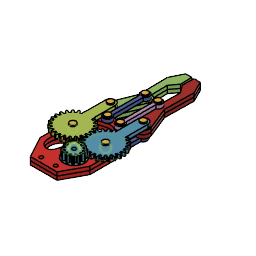
ARC Robotic-Gripper (Autodesk Fusion 360 design; units mm, degrees)
part number: 2026-08-30-15-38-19-867
part number: 2026-08-30-16-06-25-196
part number: 2026-08-30-16-15-02-917
part number: 2026-08-30-20-55-51-300
description: Spur Gear; Module: 1.125; Num Teeth: 24; Pressure Angle: 20.0; Backlash: 0.00 mm
part number: 2026-08-30-21-05-14-429
part number: 2026-08-30-21-11-26-364
part number: 2026-08-30-22-11-41-615
description: Spur Gear; Module: 1.1; Num Teeth: 12; Pressure Angle: 20.0; Backlash: 0.00 mm
part number: 2026-08-30-22-17-12-966
Autodesk Fusion 360 part; units mm, degrees
note: some values were not read from the file. Chosen so that the rebuilt part matches the saved one: a direction. Set by a fixed rule: which sketch regions a step uses.
(part 1 of 8)
sketch "Sketch1" plane through (0, 0, 0) normal (0, 1, 0) x (1, 0, 0)
  line L0 (0, -5) -> (22, -5)
  arc A0 (22, -5) -> (22, 5) centre (22, 0) ccw
  line L1 (22, 5) -> (0, 5)
  arc A1 (0, 5) -> (0, -5) centre (0, 0) ccw
  line L2 (0, 0) -> (22, 0) construction
  circle A2 centre (0, 0) radius 1.5
  line L3 (20.05, 5) -> (51.3472, 18.2849)
  line L4 (51.3472, 18.2849) -> (55.3871, 8.7674)
  line L5 (55.3871, 8.7674) -> (24.4042, -4.384)
  line L6 (42.1568, 14.3838) -> (53.3671, 13.5261)
  line L7 (26.6766, 1.769) -> (39, 7)
  line L8 (39, 7) -> (46.5562, 5.0189)
  circle A3 centre (22, 0) radius 1.5
  dimension "d1" = 22
  dimension "d2" = 5
  dimension "d3" = 3
  dimension "d4" = 157
  dimension "d5" = 34
  dimension "d6" = 1.95
  dimension "d7" = 3
  constraint tangent L0 A0
  constraint tangent A0 L1
  constraint parallel L0 L1
  constraint tangent L1 A1
  constraint tangent L0 A1
  constraint horizontal L2
  constraint coincident A1.centre L2.start
  constraint coincident L1 L3.start
  constraint perpendicular L3 L4
  constraint coincident A0 L5.end
  constraint perpendicular L4 L5
  constraint coincident L3 L6.start
  constraint midpoint L4 L6.end
  constraint coincident A0 L7.start
  constraint perpendicular L4 L7
  constraint coincident L5 L8.end
  constraint concentric A0 A3
  measures "d1" distance of A1.centre A0.centre
  measures "d2" radius of A1
  measures "d3" diameter of A2
  measures "d4" angle of L1 L3
  measures "d5" distance of L3.start L3.end
  measures "d6" horizontal distance of A0.centre L3.start
  measures "d7" diameter of A3
extrude "Extrude1" add sketch "Sketch1" along normal blind 3 contours L0 A0 L1 A1 | A0 L1 L3 L4 L5 L6 L7 L8 makes body 1
copy_body "Body->Comp1" bodies 1 removing the originals makes body 2 in component "Component"
sketch "Sketch2" plane through (0, 0, 0) normal (0, 1, 0) x (1, 0, 0)
  circle A0 centre (2, 10) radius 1.5
  circle A1 centre (2, 10) radius 3.5
  circle A2 centre (33, 10) radius 3.5
  circle A3 centre (33, 10) radius 1.5
  line L0 (2, 10) -> (33, 10)
  line L1 (5.1623, 11.5) -> (29.8377, 11.5)
  line L2 (5.1623, 8.5) -> (29.8377, 8.5)
  dimension "d11" = 7
  dimension "d12" = 3
  dimension "d14" = 7
  dimension "d15" = 3
  dimension "d16" = 31
  dimension "d17" = 1.5
  constraint concentric A0 A1
  constraint concentric A2 A3
  constraint coincident A0.centre A1.centre
  constraint coincident A2.centre A3.centre
  constraint horizontal L0
  constraint coincident A1 L1.start
  constraint coincident A2 L1.end
  constraint parallel L0 L1
  constraint symmetric L0 L1.start L2.start
  constraint symmetric L0 L1.end L2.end
  measures "d11" diameter of A1
  measures "d12" diameter of A0
  measures "d14" diameter of A2
  measures "d15" diameter of A3
  measures "d16" distance of A0.centre A2.centre
  measures "d17" distance of L0 L1
extrude "Extrude1'" add sketch "Sketch2" along normal blind 3 separate body makes body 3 in component "Component'"
sketch "Sketch3" plane through (0, 0, 0) normal (0, 1, 0) x (1, 0, 0)
  line L0 (0, 0) -> (0, 62) construction
  line L1 (0, 62) -> (-7.9898, 62)
  line L2 (-7.9898, 62) -> (-20.5, 47.8997)
  line L3 (-20.5, 47.8997) -> (-20.5, 17.5997)
  line L4 (-20.5, 17.5997) -> (-11, 0)
  line L5 (-11, 0) -> (0, 0)
  circle A0 centre (-6, 4) radius 1.5
  circle A1 centre (-13.5, 37.5997) radius 1.5
  circle A2 centre (-5.2398, 58) radius 1.5
  circle A3 centre (6, 4) radius 1.5
  line L6 (20.5, 47.8997) -> (20.5, 17.5997)
  circle A4 centre (5.2398, 58) radius 1.5
  circle A5 centre (13.5, 37.5997) radius 1.5
  line L7 (20.5, 17.5997) -> (11, 0)
  line L8 (11, 0) -> (0, 0)
  line L9 (0, 62) -> (7.9898, 62)
  line L10 (7.9898, 62) -> (20.5, 47.8997)
  circle A6 centre (7.5, 17.5997) radius 8.5
  line L11 (20.5, 17.5997) -> (2, 17.5997) construction
  dimension "d20" = 62
  dimension "d21" = 11
  dimension "d22" = 20
  dimension "d23" = 20.5
  dimension "d24" = 30.3
  dimension "d25" = 18.85
  dimension "d26" = 3
  dimension "d27" = 3
  dimension "d28" = 3
  dimension "d29" = 4
  dimension "d30" = 2.75
  dimension "d31" = 10.3
  dimension "d32" = 7
  dimension "d33" = 6
  dimension "d34" = 4
  dimension "d35" = 17
  dimension "d36" = 13
  constraint coincident L0.start L5.end
  constraint vertical L0
  constraint perpendicular L0 L1
  constraint perpendicular L1 L3
  constraint perpendicular L0 L5
  constraint symmetric L5.end L0 L8.end
  constraint symmetric L1.start L0 L9.start
  constraint symmetric L0 L1.end L9.end
  constraint symmetric L0 L2.end L6.start
  constraint symmetric L0 L3.end L6.end
  constraint symmetric L0 L4.end L7.end
  constraint symmetric L0 A0 A3
  constraint symmetric L0 A1 A5
  constraint symmetric L0 A2 A4
  constraint perpendicular L6 L11
  measures "d20" distance of L0.start L0.end
  measures "d21" distance of L0.start L4.end
  measures "d22" distance of L3.end L4.end
  measures "d23" distance of L0 L3
  measures "d24" distance of L2.end L3.end
  measures "d25" distance of L1.end L2.end
  measures "d26" diameter of A0
  measures "d27" diameter of A1
  measures "d28" diameter of A2
  measures "d29" distance of L1 A2.centre
  measures "d30" horizontal distance of L1.end A2.centre
  measures "d31" vertical distance of L2.end A1.centre
  measures "d32" distance of L3 A1.centre
  measures "d33" distance of L0 A0.centre
  measures "d34" distance of L5 A0.centre
  measures "d35" diameter of A6
  measures "d36" distance of L6.end A6.centre
extrude "Extrude1''" add sketch "Sketch3" along normal blind 3 separate body makes body 4 in component "Component''"
sketch "Sketch4" plane through (0, 3, 0) normal (0, 1, 0) x (-1, 0, 0)
  circle A0 centre (13.5, -37.5997) radius 1.5
  circle A1 centre (-13.5, -37.5997) radius 1.5
  circle A2 centre (5.2398, -58) radius 1.5
  circle A3 centre (-5.2398, -58) radius 1.5
  circle A4 centre (-7.5, -17.5997) radius 8.5
  circle A5 centre (-6, -4) radius 1.5
  circle A6 centre (6, -4) radius 1.5
  line L0 (-7.9898, -62) -> (7.9898, -62)
  line L1 (7.9898, -62) -> (20.5, -47.8997)
  line L2 (20.5, -47.8997) -> (20.5, -17.5997)
  line L3 (20.5, -17.5997) -> (11, 0)
  line L4 (11, 0) -> (-11, 0)
  line L5 (-11, 0) -> (-20.5, -17.5997)
  line L6 (-20.5, -17.5997) -> (-20.5, -47.8997)
  line L7 (-20.5, -47.8997) -> (-7.9898, -62)
  spline S0 degree 5 poles (-5.4336, -53.3907) (-5.0466, -53.6541) (-4.2829, -54.1428) (-3.1766, -54.7552) (-1.7949, -55.3213) (-0.1877, -55.6395) (1.3743, -55.6316) (2.9743, -55.3768) (4.672, -54.9534) (6.4712, -54.4196) (8.2906, -53.797) (9.9982, -53.0839) (11.4425, -52.2666) (12.4861, -51.3325) (13.0351, -50.2808) (13.0781, -49.1379) (12.6944, -47.958) (12.0103, -46.799) (11.1693, -45.705) (10.2934, -44.6837) (9.4576, -43.6945) (8.7075, -42.6752) (8.0713, -41.564) (7.5718, -40.321) (7.2426, -38.9561) (7.1252, -37.5229) (7.2563, -36.0942) (7.6582, -34.7424) (8.3281, -33.5194) (9.2262, -32.434) (10.2859, -31.4594) (11.4259, -30.5457) (12.5628, -29.6303) (13.6225, -28.649) (14.5534, -27.5475) (15.3216, -26.2861) (15.9046, -24.8443) (16.2852, -23.226) (16.4461, -21.4627) (16.3624, -19.621) (16.0068, -17.7946) (15.3609, -16.0912) (14.4242, -14.6215) (13.2244, -13.4867) (11.8261, -12.7674) (10.3439, -12.5104) (8.9154, -12.7294) (7.6684, -13.407) (6.6915, -14.497) (5.9989, -15.9255) (5.5123, -17.5946) (5.1029, -19.3938) (4.6229, -21.2096) (3.9421, -22.9364) (2.9802, -24.4864) (1.7452, -25.8008) (0.3576, -26.858) (-1.0142, -27.6679) (-2.2075, -28.2677) (-3.1243, -28.7169) (-3.7864, -29.0927) (-4.3954, -29.4854) (-5.191, -29.9812) (-6.3187, -30.6456) (-7.6675, -31.5043) (-8.9566, -32.5465) (-9.8678, -33.7315) (-10.1614, -34.9951) (-9.7992, -36.2553) (-9.0659, -37.4185) (-8.3987, -38.4052) (-8.218, -39.1757) (-8.7535, -39.7561) (-9.8832, -40.2621) (-11.2724, -40.8519) (-12.505, -41.6801) (-13.2098, -42.8549) (-13.2068, -44.3863) (-12.4853, -46.202) (-11.1517, -48.176) (-9.3881, -50.1522) (-7.8027, -51.6062) (-6.6047, -52.5623) (-5.8205, -53.1273) (-5.4336, -53.3907) knots 0 0 0 0 0 0 0.0125 0.025 0.0375 0.05 0.0625 0.075 0.0875 0.1 0.1125 0.125 0.1375 0.15 0.1625 0.175 0.1875 0.2 0.2125 0.225 0.2375 0.25 0.2625 0.275 0.2875 0.3 0.3125 0.325 0.3375 0.35 0.3625 0.375 0.3875 0.4 0.4125 0.425 0.4375 0.45 0.4625 0.475 0.4875 0.5 0.5125 0.525 0.5375 0.55 0.5625 0.575 0.5875 0.6 0.6125 0.625 0.6375 0.65 0.6625 0.675 0.6875 0.7 0.7125 0.725 0.7375 0.75 0.7625 0.775 0.7875 0.8 0.8125 0.825 0.8375 0.85 0.8625 0.875 0.8875 0.9 0.9125 0.925 0.9375 0.95 0.9625 0.975 0.9875 1 1 1 1 1 1
  point P0 (4.6067, -54.9499)
  point P1 (12.7571, -50.674)
  point P2 (11.3396, -45.9491)
  point P3 (7.9141, -41.1061)
  point P4 (7.796, -34.6095)
  point P5 (12.639, -29.5303)
  point P6 (16.3007, -22.6793)
  point P7 (12.9933, -13.4658)
  point P8 (6.9691, -14.2927)
  point P9 (3.0711, -24.2148)
  point P10 (-3.0711, -28.7034)
  point P11 (-5.4336, -30.1209)
  point P12 (-10, -35)
  point P13 (-8.3866, -39.0981)
  point P14 (-12.5208, -41.933)
extrude "Extrude2" cut sketch "Sketch4" against normal blind 5 contours S0 bodies 4 in component "Component''"
sketch "Base Circle" plane through (0, 0, 0) normal (0, 0, 1) x (1, 0, 0) in component "Spur Gear 24 teeth"
  circle A0 centre (0, 0) radius 12.1984
  circle A1 centre (0, 0) radius 1.5
extrude "Extrude1'''" add sketch "Base Circle" along normal blind 3 separate body makes body 5 in component "Spur Gear 24 teeth"
sketch "Gear Tooth" plane through (0, 0, 0) normal (0, 0, 1) x (1, 0, 0) in component "Spur Gear 24 teeth"
  spline S0 degree 5 poles (12.6449, -1.0183) (12.6506, -1.0187) (12.6618, -1.0195) (12.6788, -1.0202) (12.7014, -1.0204) (12.7297, -1.0195) (12.758, -1.0178) (12.7864, -1.0156) (12.8147, -1.0131) (12.8431, -1.0105) (12.8715, -1.0076) (12.8999, -1.0045) (12.9284, -1.0011) (12.9568, -0.9973) (12.9852, -0.9932) (13.0137, -0.9886) (13.0421, -0.9838) (13.0705, -0.9787) (13.099, -0.9733) (13.1274, -0.9678) (13.1559, -0.962) (13.1843, -0.956) (13.2127, -0.9498) (13.2412, -0.9433) (13.2696, -0.9366) (13.298, -0.9297) (13.3264, -0.9226) (13.3549, -0.9152) (13.3833, -0.9076) (13.4117, -0.8999) (13.4401, -0.8919) (13.4684, -0.8838) (13.4968, -0.8754) (13.5252, -0.8669) (13.5535, -0.8581) (13.5819, -0.8492) (13.6102, -0.8401) (13.6385, -0.8308) (13.6669, -0.8214) (13.6952, -0.8117) (13.7234, -0.8019) (13.7517, -0.7919) (13.78, -0.7817) (13.8082, -0.7714) (13.8365, -0.7609) (13.8647, -0.7502) (13.8929, -0.7393) (13.9211, -0.7283) (13.9492, -0.7171) (13.9774, -0.7058) (14.0055, -0.6943) (14.0337, -0.6826) (14.0618, -0.6708) (14.0898, -0.6588) (14.1179, -0.6467) (14.146, -0.6344) (14.174, -0.6219) (14.202, -0.6093) (14.23, -0.5966) (14.2579, -0.5837) (14.2859, -0.5706) (14.3138, -0.5574) (14.3417, -0.544) (14.3696, -0.5305) (14.3975, -0.5169) (14.4253, -0.5031) (14.4531, -0.4891) (14.4809, -0.4751) (14.5087, -0.4608) (14.5364, -0.4465) (14.5641, -0.4319) (14.5863, -0.4202) (14.6029, -0.4114) (14.6139, -0.4054) (14.6195, -0.4024) knots 0 0 0 0 0 0 0.01428571 0.02857143 0.04285714 0.05714286 0.07142857 0.08571429 0.1 0.11428571 0.12857143 0.14285714 0.15714286 0.17142857 0.18571429 0.2 0.21428571 0.22857143 0.24285714 0.25714286 0.27142857 0.28571429 0.3 0.31428571 0.32857143 0.34285714 0.35714286 0.37142857 0.38571429 0.4 0.41428571 0.42857143 0.44285714 0.45714286 0.47142857 0.48571429 0.5 0.51428571 0.52857143 0.54285714 0.55714286 0.57142857 0.58571429 0.6 0.61428571 0.62857143 0.64285714 0.65714286 0.67142857 0.68571429 0.7 0.71428571 0.72857143 0.74285714 0.75714286 0.77142857 0.78571429 0.8 0.81428571 0.82857143 0.84285714 0.85714286 0.87142857 0.88571429 0.9 0.91428571 0.92857143 0.94285714 0.95714286 0.97142857 0.98571429 1 1 1 1 1 1
  spline S1 degree 5 poles (12.6449, 1.0183) (12.6506, 1.0187) (12.6618, 1.0195) (12.6788, 1.0202) (12.7014, 1.0204) (12.7297, 1.0195) (12.758, 1.0178) (12.7864, 1.0156) (12.8147, 1.0131) (12.8431, 1.0105) (12.8715, 1.0076) (12.8999, 1.0045) (12.9284, 1.0011) (12.9568, 0.9973) (12.9852, 0.9932) (13.0137, 0.9886) (13.0421, 0.9838) (13.0705, 0.9787) (13.099, 0.9733) (13.1274, 0.9678) (13.1559, 0.962) (13.1843, 0.956) (13.2127, 0.9498) (13.2412, 0.9433) (13.2696, 0.9366) (13.298, 0.9297) (13.3264, 0.9226) (13.3549, 0.9152) (13.3833, 0.9076) (13.4117, 0.8999) (13.4401, 0.8919) (13.4684, 0.8838) (13.4968, 0.8754) (13.5252, 0.8669) (13.5535, 0.8581) (13.5819, 0.8492) (13.6102, 0.8401) (13.6385, 0.8308) (13.6669, 0.8214) (13.6952, 0.8117) (13.7234, 0.8019) (13.7517, 0.7919) (13.78, 0.7817) (13.8082, 0.7714) (13.8365, 0.7609) (13.8647, 0.7502) (13.8929, 0.7393) (13.9211, 0.7283) (13.9492, 0.7171) (13.9774, 0.7058) (14.0055, 0.6943) (14.0337, 0.6826) (14.0618, 0.6708) (14.0898, 0.6588) (14.1179, 0.6467) (14.146, 0.6344) (14.174, 0.6219) (14.202, 0.6093) (14.23, 0.5966) (14.2579, 0.5837) (14.2859, 0.5706) (14.3138, 0.5574) (14.3417, 0.544) (14.3696, 0.5305) (14.3975, 0.5169) (14.4253, 0.5031) (14.4531, 0.4891) (14.4809, 0.4751) (14.5087, 0.4608) (14.5364, 0.4465) (14.5641, 0.4319) (14.5863, 0.4202) (14.6029, 0.4114) (14.6139, 0.4054) (14.6195, 0.4024) knots 0 0 0 0 0 0 0.01428571 0.02857143 0.04285714 0.05714286 0.07142857 0.08571429 0.1 0.11428571 0.12857143 0.14285714 0.15714286 0.17142857 0.18571429 0.2 0.21428571 0.22857143 0.24285714 0.25714286 0.27142857 0.28571429 0.3 0.31428571 0.32857143 0.34285714 0.35714286 0.37142857 0.38571429 0.4 0.41428571 0.42857143 0.44285714 0.45714286 0.47142857 0.48571429 0.5 0.51428571 0.52857143 0.54285714 0.55714286 0.57142857 0.58571429 0.6 0.61428571 0.62857143 0.64285714 0.65714286 0.67142857 0.68571429 0.7 0.71428571 0.72857143 0.74285714 0.75714286 0.77142857 0.78571429 0.8 0.81428571 0.82857143 0.84285714 0.85714286 0.87142857 0.88571429 0.9 0.91428571 0.92857143 0.94285714 0.95714286 0.97142857 0.98571429 1 1 1 1 1 1
  arc A0 (14.6195, -0.4024) -> (14.6195, 0.4024) centre (0, 0) ccw
  line L0 (12.149, -0.9783) -> (12.6449, -1.0183)
  line L1 (12.149, 0.9783) -> (12.6449, 1.0183)
  line L2 (12.149, -0.9783) -> (12.149, 0.9783)
  point P0 (12.7841, -1.0157)
  point P1 (12.9241, -1.0016)
  point P2 (13.0647, -0.9797)
  point P3 (13.2057, -0.9513)
  point P4 (13.3469, -0.9172)
  point P5 (13.4884, -0.8779)
  point P6 (13.63, -0.8336)
  point P7 (13.7716, -0.7847)
  point P8 (13.9132, -0.7313)
  point P9 (14.0548, -0.6737)
  point P10 (14.1963, -0.6119)
  point P11 (14.3376, -0.546)
  point P12 (14.4787, -0.4761)
  point P13 (12.7841, 1.0157)
  point P14 (12.9241, 1.0016)
  point P15 (13.0647, 0.9797)
  point P16 (13.2057, 0.9513)
  point P17 (13.3469, 0.9172)
  point P18 (13.4884, 0.8779)
  point P19 (13.63, 0.8336)
  point P20 (13.7716, 0.7847)
  point P21 (13.9132, 0.7313)
  point P22 (14.0548, 0.6737)
  point P23 (14.1963, 0.6119)
  point P24 (14.3376, 0.546)
  point P25 (14.4787, 0.4761)
extrude "Extrude2'" add sketch "Gear Tooth" along normal blind 3 bodies 5 in component "Spur Gear 24 teeth"
fillet "Fillet1" radius 0.1 2 edges at (12.159, -0.9791, 1.5) (12.159, 0.9791, 1.5) on bodies 5 in component "Spur Gear 24 teeth"
pattern_circular "C-Pattern1" count 24 over 360 about axis through (0, 0, 0) along (0, 0, 1) of "Extrude2'", "Fillet1" in component "Spur Gear 24 teeth"
sketch "Diametrial Pitch Circle" plane through (0, 0, 0) normal (0, 0, 1) x (1, 0, 0) in component "Spur Gear 24 teeth"
  circle A0 centre (0, 0) radius 13.5 construction
sketch "Base Circle (2)" plane through (0, 0, 0) normal (0, 0, 1) x (1, 0, 0) in component "Spur Gear 24 teeth (1)"
  circle A0 centre (0, 0) radius 12.1984
  circle A1 centre (0, 0) radius 1.5
extrude "Extrude1''''" add sketch "Base Circle (2)" along normal blind 3 separate body makes body 6 in component "Spur Gear 24 teeth (1)"
sketch "Gear Tooth (2)" plane through (0, 0, 0) normal (0, 0, 1) x (1, 0, 0) in component "Spur Gear 24 teeth (1)"
  spline S0 degree 5 poles (12.6449, -1.0183) (12.6506, -1.0187) (12.6618, -1.0195) (12.6788, -1.0202) (12.7014, -1.0204) (12.7297, -1.0195) (12.758, -1.0178) (12.7864, -1.0156) (12.8147, -1.0131) (12.8431, -1.0105) (12.8715, -1.0076) (12.8999, -1.0045) (12.9284, -1.0011) (12.9568, -0.9973) (12.9852, -0.9932) (13.0137, -0.9886) (13.0421, -0.9838) (13.0705, -0.9787) (13.099, -0.9733) (13.1274, -0.9678) (13.1559, -0.962) (13.1843, -0.956) (13.2127, -0.9498) (13.2412, -0.9433) (13.2696, -0.9366) (13.298, -0.9297) (13.3264, -0.9226) (13.3549, -0.9152) (13.3833, -0.9076) (13.4117, -0.8999) (13.4401, -0.8919) (13.4684, -0.8838) (13.4968, -0.8754) (13.5252, -0.8669) (13.5535, -0.8581) (13.5819, -0.8492) (13.6102, -0.8401) (13.6385, -0.8308) (13.6669, -0.8214) (13.6952, -0.8117) (13.7234, -0.8019) (13.7517, -0.7919) (13.78, -0.7817) (13.8082, -0.7714) (13.8365, -0.7609) (13.8647, -0.7502) (13.8929, -0.7393) (13.9211, -0.7283) (13.9492, -0.7171) (13.9774, -0.7058) (14.0055, -0.6943) (14.0337, -0.6826) (14.0618, -0.6708) (14.0898, -0.6588) (14.1179, -0.6467) (14.146, -0.6344) (14.174, -0.6219) (14.202, -0.6093) (14.23, -0.5966) (14.2579, -0.5837) (14.2859, -0.5706) (14.3138, -0.5574) (14.3417, -0.544) (14.3696, -0.5305) (14.3975, -0.5169) (14.4253, -0.5031) (14.4531, -0.4891) (14.4809, -0.4751) (14.5087, -0.4608) (14.5364, -0.4465) (14.5641, -0.4319) (14.5863, -0.4202) (14.6029, -0.4114) (14.6139, -0.4054) (14.6195, -0.4024) knots 0 0 0 0 0 0 0.01428571 0.02857143 0.04285714 0.05714286 0.07142857 0.08571429 0.1 0.11428571 0.12857143 0.14285714 0.15714286 0.17142857 0.18571429 0.2 0.21428571 0.22857143 0.24285714 0.25714286 0.27142857 0.28571429 0.3 0.31428571 0.32857143 0.34285714 0.35714286 0.37142857 0.38571429 0.4 0.41428571 0.42857143 0.44285714 0.45714286 0.47142857 0.48571429 0.5 0.51428571 0.52857143 0.54285714 0.55714286 0.57142857 0.58571429 0.6 0.61428571 0.62857143 0.64285714 0.65714286 0.67142857 0.68571429 0.7 0.71428571 0.72857143 0.74285714 0.75714286 0.77142857 0.78571429 0.8 0.81428571 0.82857143 0.84285714 0.85714286 0.87142857 0.88571429 0.9 0.91428571 0.92857143 0.94285714 0.95714286 0.97142857 0.98571429 1 1 1 1 1 1
  spline S1 degree 5 poles (12.6449, 1.0183) (12.6506, 1.0187) (12.6618, 1.0195) (12.6788, 1.0202) (12.7014, 1.0204) (12.7297, 1.0195) (12.758, 1.0178) (12.7864, 1.0156) (12.8147, 1.0131) (12.8431, 1.0105) (12.8715, 1.0076) (12.8999, 1.0045) (12.9284, 1.0011) (12.9568, 0.9973) (12.9852, 0.9932) (13.0137, 0.9886) (13.0421, 0.9838) (13.0705, 0.9787) (13.099, 0.9733) (13.1274, 0.9678) (13.1559, 0.962) (13.1843, 0.956) (13.2127, 0.9498) (13.2412, 0.9433) (13.2696, 0.9366) (13.298, 0.9297) (13.3264, 0.9226) (13.3549, 0.9152) (13.3833, 0.9076) (13.4117, 0.8999) (13.4401, 0.8919) (13.4684, 0.8838) (13.4968, 0.8754) (13.5252, 0.8669) (13.5535, 0.8581) (13.5819, 0.8492) (13.6102, 0.8401) (13.6385, 0.8308) (13.6669, 0.8214) (13.6952, 0.8117) (13.7234, 0.8019) (13.7517, 0.7919) (13.78, 0.7817) (13.8082, 0.7714) (13.8365, 0.7609) (13.8647, 0.7502) (13.8929, 0.7393) (13.9211, 0.7283) (13.9492, 0.7171) (13.9774, 0.7058) (14.0055, 0.6943) (14.0337, 0.6826) (14.0618, 0.6708) (14.0898, 0.6588) (14.1179, 0.6467) (14.146, 0.6344) (14.174, 0.6219) (14.202, 0.6093) (14.23, 0.5966) (14.2579, 0.5837) (14.2859, 0.5706) (14.3138, 0.5574) (14.3417, 0.544) (14.3696, 0.5305) (14.3975, 0.5169) (14.4253, 0.5031) (14.4531, 0.4891) (14.4809, 0.4751) (14.5087, 0.4608) (14.5364, 0.4465) (14.5641, 0.4319) (14.5863, 0.4202) (14.6029, 0.4114) (14.6139, 0.4054) (14.6195, 0.4024) knots 0 0 0 0 0 0 0.01428571 0.02857143 0.04285714 0.05714286 0.07142857 0.08571429 0.1 0.11428571 0.12857143 0.14285714 0.15714286 0.17142857 0.18571429 0.2 0.21428571 0.22857143 0.24285714 0.25714286 0.27142857 0.28571429 0.3 0.31428571 0.32857143 0.34285714 0.35714286 0.37142857 0.38571429 0.4 0.41428571 0.42857143 0.44285714 0.45714286 0.47142857 0.48571429 0.5 0.51428571 0.52857143 0.54285714 0.55714286 0.57142857 0.58571429 0.6 0.61428571 0.62857143 0.64285714 0.65714286 0.67142857 0.68571429 0.7 0.71428571 0.72857143 0.74285714 0.75714286 0.77142857 0.78571429 0.8 0.81428571 0.82857143 0.84285714 0.85714286 0.87142857 0.88571429 0.9 0.91428571 0.92857143 0.94285714 0.95714286 0.97142857 0.98571429 1 1 1 1 1 1
  arc A0 (14.6195, -0.4024) -> (14.6195, 0.4024) centre (0, 0) ccw
  line L0 (12.149, -0.9783) -> (12.6449, -1.0183)
  line L1 (12.149, 0.9783) -> (12.6449, 1.0183)
  line L2 (12.149, -0.9783) -> (12.149, 0.9783)
  point P0 (12.7841, -1.0157)
  point P1 (12.9241, -1.0016)
  point P2 (13.0647, -0.9797)
  point P3 (13.2057, -0.9513)
  point P4 (13.3469, -0.9172)
  point P5 (13.4884, -0.8779)
  point P6 (13.63, -0.8336)
  point P7 (13.7716, -0.7847)
  point P8 (13.9132, -0.7313)
  point P9 (14.0548, -0.6737)
  point P10 (14.1963, -0.6119)
  point P11 (14.3376, -0.546)
  point P12 (14.4787, -0.4761)
  point P13 (12.7841, 1.0157)
  point P14 (12.9241, 1.0016)
  point P15 (13.0647, 0.9797)
  point P16 (13.2057, 0.9513)
  point P17 (13.3469, 0.9172)
  point P18 (13.4884, 0.8779)
  point P19 (13.63, 0.8336)
  point P20 (13.7716, 0.7847)
  point P21 (13.9132, 0.7313)
  point P22 (14.0548, 0.6737)
  point P23 (14.1963, 0.6119)
  point P24 (14.3376, 0.546)
  point P25 (14.4787, 0.4761)
extrude "Extrude2''" add sketch "Gear Tooth (2)" along normal blind 3 bodies 6 in component "Spur Gear 24 teeth (1)"
fillet "Fillet1'" radius 0.1 2 edges at (12.159, -0.9791, 1.5) (12.159, 0.9791, 1.5) on bodies 6 in component "Spur Gear 24 teeth (1)"
pattern_circular "C-Pattern1'" count 24 over 360 about axis through (0, 0, 0) along (0, 0, 1) of "Extrude2''", "Fillet1'" in component "Spur Gear 24 teeth (1)"
sketch "Diametrial Pitch Circle (2)" plane through (0, 0, 0) normal (0, 0, 1) x (1, 0, 0) in component "Spur Gear 24 teeth (1)"
  circle A0 centre (0, 0) radius 13.5 construction
sketch "Sketch5" plane through (0, 6, 0) normal (0, 1, 0) x (-1, 0, 0)
  arc A0 (11.3964, -49.6153) -> (12.422, -49.7504) centre (13.5, -37.5997) ccw
  arc A1 (12.5129, -49.858) -> (12.422, -49.7504) centre (12.4132, -49.85) ccw
  line L0 (12.5129, -49.858) -> (12.4817, -50.2446)
  spline S0 degree 5 poles (12.4817, -50.2446) (12.4813, -50.2503) (12.4805, -50.2616) (12.4798, -50.2785) (12.4796, -50.3011) (12.4805, -50.3294) (12.4822, -50.3577) (12.4844, -50.3861) (12.4869, -50.4145) (12.4895, -50.4429) (12.4924, -50.4713) (12.4955, -50.4997) (12.4989, -50.5281) (12.5027, -50.5565) (12.5068, -50.5849) (12.5114, -50.6134) (12.5162, -50.6418) (12.5213, -50.6703) (12.5267, -50.6987) (12.5322, -50.7271) (12.538, -50.7556) (12.544, -50.784) (12.5502, -50.8124) (12.5567, -50.8409) (12.5634, -50.8693) (12.5703, -50.8977) (12.5774, -50.9262) (12.5848, -50.9546) (12.5924, -50.983) (12.6001, -51.0114) (12.6081, -51.0398) (12.6162, -51.0682) (12.6246, -51.0965) (12.6331, -51.1249) (12.6419, -51.1533) (12.6508, -51.1816) (12.6599, -51.2099) (12.6692, -51.2383) (12.6786, -51.2666) (12.6883, -51.2949) (12.6981, -51.3232) (12.7081, -51.3514) (12.7183, -51.3797) (12.7286, -51.4079) (12.7391, -51.4362) (12.7498, -51.4644) (12.7607, -51.4926) (12.7717, -51.5208) (12.7829, -51.549) (12.7942, -51.5771) (12.8057, -51.6052) (12.8174, -51.6334) (12.8292, -51.6615) (12.8412, -51.6896) (12.8533, -51.7176) (12.8656, -51.7457) (12.8781, -51.7737) (12.8907, -51.8017) (12.9034, -51.8297) (12.9163, -51.8577) (12.9294, -51.8856) (12.9426, -51.9135) (12.956, -51.9414) (12.9695, -51.9693) (12.9831, -51.9972) (12.9969, -52.025) (13.0109, -52.0528) (13.0249, -52.0806) (13.0392, -52.1084) (13.0535, -52.1361) (13.0681, -52.1638) (13.0798, -52.186) (13.0886, -52.2026) (13.0946, -52.2136) (13.0976, -52.2192) knots 0 0 0 0 0 0 0.01428571 0.02857143 0.04285714 0.05714286 0.07142857 0.08571429 0.1 0.11428571 0.12857143 0.14285714 0.15714286 0.17142857 0.18571429 0.2 0.21428571 0.22857143 0.24285714 0.25714286 0.27142857 0.28571429 0.3 0.31428571 0.32857143 0.34285714 0.35714286 0.37142857 0.38571429 0.4 0.41428571 0.42857143 0.44285714 0.45714286 0.47142857 0.48571429 0.5 0.51428571 0.52857143 0.54285714 0.55714286 0.57142857 0.58571429 0.6 0.61428571 0.62857143 0.64285714 0.65714286 0.67142857 0.68571429 0.7 0.71428571 0.72857143 0.74285714 0.75714286 0.77142857 0.78571429 0.8 0.81428571 0.82857143 0.84285714 0.85714286 0.87142857 0.88571429 0.9 0.91428571 0.92857143 0.94285714 0.95714286 0.97142857 0.98571429 1 1 1 1 1 1
  arc A2 (13.0976, -52.2192) -> (13.9024, -52.2192) centre (13.5, -37.5997) ccw
  spline S1 degree 5 poles (13.9024, -52.2192) (13.9054, -52.2136) (13.9114, -52.2026) (13.9202, -52.186) (13.9319, -52.1638) (13.9465, -52.1361) (13.9608, -52.1084) (13.9751, -52.0806) (13.9891, -52.0528) (14.0031, -52.025) (14.0169, -51.9972) (14.0305, -51.9693) (14.044, -51.9414) (14.0574, -51.9135) (14.0706, -51.8856) (14.0837, -51.8577) (14.0966, -51.8297) (14.1093, -51.8017) (14.1219, -51.7737) (14.1344, -51.7457) (14.1467, -51.7176) (14.1588, -51.6896) (14.1708, -51.6615) (14.1826, -51.6334) (14.1943, -51.6052) (14.2058, -51.5771) (14.2171, -51.549) (14.2283, -51.5208) (14.2393, -51.4926) (14.2502, -51.4644) (14.2609, -51.4362) (14.2714, -51.4079) (14.2817, -51.3797) (14.2919, -51.3514) (14.3019, -51.3232) (14.3117, -51.2949) (14.3214, -51.2666) (14.3308, -51.2383) (14.3401, -51.2099) (14.3492, -51.1816) (14.3581, -51.1533) (14.3669, -51.1249) (14.3754, -51.0965) (14.3838, -51.0682) (14.3919, -51.0398) (14.3999, -51.0114) (14.4076, -50.983) (14.4152, -50.9546) (14.4226, -50.9262) (14.4297, -50.8977) (14.4366, -50.8693) (14.4433, -50.8409) (14.4498, -50.8124) (14.456, -50.784) (14.462, -50.7556) (14.4678, -50.7271) (14.4733, -50.6987) (14.4787, -50.6703) (14.4838, -50.6418) (14.4886, -50.6134) (14.4932, -50.5849) (14.4973, -50.5565) (14.5011, -50.5281) (14.5045, -50.4997) (14.5076, -50.4713) (14.5105, -50.4429) (14.5131, -50.4145) (14.5156, -50.3861) (14.5178, -50.3577) (14.5195, -50.3294) (14.5204, -50.3011) (14.5202, -50.2785) (14.5195, -50.2616) (14.5187, -50.2503) (14.5183, -50.2446) knots -1 -1 -1 -1 -1 -1 -0.98571429 -0.97142857 -0.95714286 -0.94285714 -0.92857143 -0.91428571 -0.9 -0.88571429 -0.87142857 -0.85714286 -0.84285714 -0.82857143 -0.81428571 -0.8 -0.78571429 -0.77142857 -0.75714286 -0.74285714 -0.72857143 -0.71428571 -0.7 -0.68571429 -0.67142857 -0.65714286 -0.64285714 -0.62857143 -0.61428571 -0.6 -0.58571429 -0.57142857 -0.55714286 -0.54285714 -0.52857143 -0.51428571 -0.5 -0.48571429 -0.47142857 -0.45714286 -0.44285714 -0.42857143 -0.41428571 -0.4 -0.38571429 -0.37142857 -0.35714286 -0.34285714 -0.32857143 -0.31428571 -0.3 -0.28571429 -0.27142857 -0.25714286 -0.24285714 -0.22857143 -0.21428571 -0.2 -0.18571429 -0.17142857 -0.15714286 -0.14285714 -0.12857143 -0.11428571 -0.1 -0.08571429 -0.07142857 -0.05714286 -0.04285714 -0.02857143 -0.01428571 0 0 0 0 0 0
  line L1 (14.5183, -50.2446) -> (14.4871, -49.858)
  arc A3 (14.578, -49.7504) -> (14.4871, -49.858) centre (14.5868, -49.85) ccw
  arc A4 (14.578, -49.7504) -> (15.6036, -49.6153) centre (13.5, -37.5997) ccw
  arc A5 (15.7192, -49.6958) -> (15.6036, -49.6153) centre (15.6208, -49.7138) ccw
  line L2 (15.7192, -49.6958) -> (15.7892, -50.0773)
  spline S2 degree 5 poles (15.7892, -50.0773) (15.7902, -50.0829) (15.7924, -50.094) (15.7961, -50.1105) (15.8018, -50.1324) (15.8099, -50.1595) (15.8189, -50.1864) (15.8284, -50.2133) (15.8381, -50.24) (15.848, -50.2668) (15.8581, -50.2935) (15.8684, -50.3201) (15.8791, -50.3467) (15.8901, -50.3731) (15.9015, -50.3995) (15.9132, -50.4258) (15.9253, -50.452) (15.9376, -50.4782) (15.9501, -50.5043) (15.9628, -50.5303) (15.9758, -50.5563) (15.9889, -50.5822) (16.0023, -50.6081) (16.0159, -50.6339) (16.0297, -50.6596) (16.0438, -50.6852) (16.058, -50.7108) (16.0725, -50.7364) (16.0871, -50.7619) (16.102, -50.7873) (16.117, -50.8127) (16.1322, -50.838) (16.1476, -50.8632) (16.1632, -50.8884) (16.179, -50.9135) (16.195, -50.9386) (16.2111, -50.9636) (16.2274, -50.9886) (16.2439, -51.0135) (16.2605, -51.0383) (16.2773, -51.0631) (16.2943, -51.0878) (16.3114, -51.1125) (16.3287, -51.1371) (16.3462, -51.1616) (16.3638, -51.1861) (16.3816, -51.2106) (16.3996, -51.2349) (16.4176, -51.2593) (16.4359, -51.2835) (16.4543, -51.3077) (16.4728, -51.3319) (16.4915, -51.3559) (16.5104, -51.38) (16.5294, -51.4039) (16.5485, -51.4278) (16.5678, -51.4517) (16.5872, -51.4755) (16.6068, -51.4992) (16.6265, -51.5229) (16.6463, -51.5465) (16.6663, -51.5701) (16.6864, -51.5936) (16.7067, -51.617) (16.7271, -51.6404) (16.7476, -51.6637) (16.7683, -51.6869) (16.7891, -51.7101) (16.81, -51.7333) (16.8311, -51.7563) (16.8522, -51.7794) (16.8693, -51.7977) (16.8822, -51.8115) (16.8908, -51.8206) (16.8951, -51.8252) knots 0 0 0 0 0 0 0.01428571 0.02857143 0.04285714 0.05714286 0.07142857 0.08571429 0.1 0.11428571 0.12857143 0.14285714 0.15714286 0.17142857 0.18571429 0.2 0.21428571 0.22857143 0.24285714 0.25714286 0.27142857 0.28571429 0.3 0.31428571 0.32857143 0.34285714 0.35714286 0.37142857 0.38571429 0.4 0.41428571 0.42857143 0.44285714 0.45714286 0.47142857 0.48571429 0.5 0.51428571 0.52857143 0.54285714 0.55714286 0.57142857 0.58571429 0.6 0.61428571 0.62857143 0.64285714 0.65714286 0.67142857 0.68571429 0.7 0.71428571 0.72857143 0.74285714 0.75714286 0.77142857 0.78571429 0.8 0.81428571 0.82857143 0.84285714 0.85714286 0.87142857 0.88571429 0.9 0.91428571 0.92857143 0.94285714 0.95714286 0.97142857 0.98571429 1 1 1 1 1 1
  arc A6 (16.8951, -51.8252) -> (17.6725, -51.6169) centre (13.5, -37.5997) ccw
  spline S3 degree 5 poles (17.6725, -51.6169) (17.674, -51.6108) (17.6768, -51.5985) (17.6811, -51.5802) (17.6867, -51.5558) (17.6935, -51.5252) (17.7002, -51.4947) (17.7068, -51.4642) (17.7132, -51.4337) (17.7195, -51.4033) (17.7256, -51.3728) (17.7316, -51.3424) (17.7374, -51.3119) (17.7431, -51.2815) (17.7486, -51.2511) (17.754, -51.2208) (17.7592, -51.1904) (17.7643, -51.1601) (17.7692, -51.1298) (17.774, -51.0995) (17.7786, -51.0692) (17.7831, -51.0389) (17.7874, -51.0087) (17.7915, -50.9785) (17.7955, -50.9483) (17.7993, -50.9182) (17.803, -50.888) (17.8065, -50.8579) (17.8099, -50.8279) (17.8131, -50.7978) (17.8161, -50.7678) (17.8189, -50.7378) (17.8216, -50.7078) (17.8241, -50.6779) (17.8264, -50.648) (17.8286, -50.6181) (17.8306, -50.5883) (17.8324, -50.5585) (17.8341, -50.5287) (17.8355, -50.499) (17.8368, -50.4693) (17.8379, -50.4397) (17.8388, -50.4101) (17.8395, -50.3805) (17.8401, -50.351) (17.8404, -50.3215) (17.8405, -50.292) (17.8405, -50.2626) (17.8403, -50.2333) (17.8398, -50.204) (17.8391, -50.1747) (17.8383, -50.1455) (17.8371, -50.1164) (17.8358, -50.0873) (17.8342, -50.0583) (17.8324, -50.0294) (17.8304, -50.0004) (17.8282, -49.9716) (17.8258, -49.9428) (17.8231, -49.9141) (17.8201, -49.8854) (17.8168, -49.8569) (17.8131, -49.8284) (17.8091, -49.8001) (17.8047, -49.7719) (17.8001, -49.7437) (17.7953, -49.7156) (17.7903, -49.6876) (17.7851, -49.6596) (17.7794, -49.6318) (17.773, -49.6042) (17.767, -49.5824) (17.7619, -49.5663) (17.7582, -49.5556) (17.7563, -49.5502) knots -1 -1 -1 -1 -1 -1 -0.98571429 -0.97142857 -0.95714286 -0.94285714 -0.92857143 -0.91428571 -0.9 -0.88571429 -0.87142857 -0.85714286 -0.84285714 -0.82857143 -0.81428571 -0.8 -0.78571429 -0.77142857 -0.75714286 -0.74285714 -0.72857143 -0.71428571 -0.7 -0.68571429 -0.67142857 -0.65714286 -0.64285714 -0.62857143 -0.61428571 -0.6 -0.58571429 -0.57142857 -0.55714286 -0.54285714 -0.52857143 -0.51428571 -0.5 -0.48571429 -0.47142857 -0.45714286 -0.44285714 -0.42857143 -0.41428571 -0.4 -0.38571429 -0.37142857 -0.35714286 -0.34285714 -0.32857143 -0.31428571 -0.3 -0.28571429 -0.27142857 -0.25714286 -0.24285714 -0.22857143 -0.21428571 -0.2 -0.18571429 -0.17142857 -0.15714286 -0.14285714 -0.12857143 -0.11428571 -0.1 -0.08571429 -0.07142857 -0.05714286 -0.04285714 -0.02857143 -0.01428571 0 0 0 0 0 0
  line L3 (17.7563, -49.5502) -> (17.6262, -49.1848)
  arc A7 (17.6861, -49.0573) -> (17.6262, -49.1848) centre (17.7204, -49.1513) ccw
  arc A8 (17.6861, -49.0573) -> (18.6418, -48.6615) centre (13.5, -37.5997) ccw
  arc A9 (18.7743, -48.7093) -> (18.6418, -48.6615) centre (18.6839, -48.7522) ccw
  line L4 (18.7743, -48.7093) -> (18.9406, -49.0597)
  spline S4 degree 5 poles (18.9406, -49.0597) (18.943, -49.0648) (18.948, -49.0749) (18.9559, -49.09) (18.967, -49.1096) (18.9819, -49.1337) (18.9976, -49.1574) (19.0137, -49.1808) (19.03, -49.2042) (19.0465, -49.2274) (19.0631, -49.2506) (19.08, -49.2737) (19.0972, -49.2966) (19.1147, -49.3193) (19.1325, -49.3418) (19.1507, -49.3642) (19.1691, -49.3864) (19.1877, -49.4085) (19.2066, -49.4304) (19.2256, -49.4523) (19.2448, -49.474) (19.2642, -49.4957) (19.2838, -49.5172) (19.3036, -49.5386) (19.3236, -49.5598) (19.3439, -49.581) (19.3643, -49.602) (19.3848, -49.623) (19.4056, -49.6438) (19.4265, -49.6645) (19.4476, -49.6851) (19.4689, -49.7056) (19.4903, -49.726) (19.5119, -49.7463) (19.5336, -49.7665) (19.5555, -49.7866) (19.5775, -49.8066) (19.5998, -49.8265) (19.6221, -49.8462) (19.6446, -49.8659) (19.6673, -49.8855) (19.6901, -49.905) (19.713, -49.9244) (19.7361, -49.9437) (19.7593, -49.9629) (19.7827, -49.982) (19.8062, -50.001) (19.8298, -50.0199) (19.8536, -50.0387) (19.8775, -50.0574) (19.9015, -50.076) (19.9257, -50.0945) (19.95, -50.1129) (19.9744, -50.1313) (19.9989, -50.1495) (20.0236, -50.1677) (20.0484, -50.1857) (20.0733, -50.2037) (20.0983, -50.2215) (20.1235, -50.2393) (20.1488, -50.257) (20.1742, -50.2745) (20.1997, -50.292) (20.2253, -50.3094) (20.2511, -50.3267) (20.277, -50.3439) (20.3029, -50.361) (20.329, -50.3781) (20.3552, -50.395) (20.3816, -50.4118) (20.408, -50.4286) (20.4292, -50.4419) (20.4452, -50.4518) (20.4559, -50.4585) (20.4612, -50.4618) knots 0 0 0 0 0 0 0.01428571 0.02857143 0.04285714 0.05714286 0.07142857 0.08571429 0.1 0.11428571 0.12857143 0.14285714 0.15714286 0.17142857 0.18571429 0.2 0.21428571 0.22857143 0.24285714 0.25714286 0.27142857 0.28571429 0.3 0.31428571 0.32857143 0.34285714 0.35714286 0.37142857 0.38571429 0.4 0.41428571 0.42857143 0.44285714 0.45714286 0.47142857 0.48571429 0.5 0.51428571 0.52857143 0.54285714 0.55714286 0.57142857 0.58571429 0.6 0.61428571 0.62857143 0.64285714 0.65714286 0.67142857 0.68571429 0.7 0.71428571 0.72857143 0.74285714 0.75714286 0.77142857 0.78571429 0.8 0.81428571 0.82857143 0.84285714 0.85714286 0.87142857 0.88571429 0.9 0.91428571 0.92857143 0.94285714 0.95714286 0.97142857 0.98571429 1 1 1 1 1 1
  arc A10 (20.4612, -50.4618) -> (21.1583, -50.0593) centre (13.5, -37.5997) ccw
  spline S5 degree 5 poles (21.1583, -50.0593) (21.1581, -50.053) (21.1577, -50.0405) (21.157, -50.0217) (21.1561, -49.9966) (21.1548, -49.9654) (21.1534, -49.9342) (21.1519, -49.903) (21.1502, -49.8719) (21.1483, -49.8408) (21.1464, -49.8098) (21.1442, -49.7789) (21.142, -49.748) (21.1396, -49.7171) (21.1371, -49.6864) (21.1344, -49.6556) (21.1316, -49.625) (21.1287, -49.5943) (21.1256, -49.5638) (21.1224, -49.5333) (21.119, -49.5028) (21.1155, -49.4725) (21.1118, -49.4422) (21.108, -49.4119) (21.104, -49.3817) (21.0999, -49.3516) (21.0957, -49.3216) (21.0913, -49.2916) (21.0867, -49.2616) (21.082, -49.2318) (21.0771, -49.202) (21.0721, -49.1723) (21.067, -49.1427) (21.0617, -49.1131) (21.0562, -49.0836) (21.0505, -49.0542) (21.0447, -49.0249) (21.0388, -48.9956) (21.0327, -48.9665) (21.0264, -48.9374) (21.0199, -48.9083) (21.0133, -48.8794) (21.0065, -48.8506) (20.9996, -48.8218) (20.9924, -48.7932) (20.9851, -48.7646) (20.9777, -48.7361) (20.97, -48.7078) (20.9622, -48.6795) (20.9542, -48.6513) (20.9459, -48.6232) (20.9375, -48.5952) (20.9289, -48.5674) (20.9201, -48.5396) (20.911, -48.512) (20.9018, -48.4845) (20.8924, -48.4571) (20.8828, -48.4298) (20.873, -48.4026) (20.863, -48.3756) (20.8527, -48.3487) (20.8421, -48.322) (20.8312, -48.2954) (20.8199, -48.2691) (20.8084, -48.243) (20.7967, -48.217) (20.7848, -48.1911) (20.7727, -48.1653) (20.7604, -48.1396) (20.7477, -48.1142) (20.7344, -48.0893) (20.7229, -48.0698) (20.7138, -48.0554) (20.7075, -48.0461) (20.7043, -48.0414) knots -1 -1 -1 -1 -1 -1 -0.98571429 -0.97142857 -0.95714286 -0.94285714 -0.92857143 -0.91428571 -0.9 -0.88571429 -0.87142857 -0.85714286 -0.84285714 -0.82857143 -0.81428571 -0.8 -0.78571429 -0.77142857 -0.75714286 -0.74285714 -0.72857143 -0.71428571 -0.7 -0.68571429 -0.67142857 -0.65714286 -0.64285714 -0.62857143 -0.61428571 -0.6 -0.58571429 -0.57142857 -0.55714286 -0.54285714 -0.52857143 -0.51428571 -0.5 -0.48571429 -0.47142857 -0.45714286 -0.44285714 -0.42857143 -0.41428571 -0.4 -0.38571429 -0.37142857 -0.35714286 -0.34285714 -0.32857143 -0.31428571 -0.3 -0.28571429 -0.27142857 -0.25714286 -0.24285714 -0.22857143 -0.21428571 -0.2 -0.18571429 -0.17142857 -0.15714286 -0.14285714 -0.12857143 -0.11428571 -0.1 -0.08571429 -0.07142857 -0.05714286 -0.04285714 -0.02857143 -0.01428571 0 0 0 0 0 0
  line L5 (20.7043, -48.0414) -> (20.484, -47.7221)
  arc A11 (20.5089, -47.5835) -> (20.484, -47.7221) centre (20.5663, -47.6653) ccw
  arc A12 (20.5089, -47.5835) -> (21.3296, -46.9538) centre (13.5, -37.5997) ccw
  arc A13 (21.4699, -46.9656) -> (21.3296, -46.9538) centre (21.3938, -47.0304) ccw
  line L6 (21.4699, -46.9656) -> (21.7213, -47.261)
  spline S6 degree 5 poles (21.7213, -47.261) (21.725, -47.2654) (21.7324, -47.2739) (21.7439, -47.2864) (21.7597, -47.3025) (21.7804, -47.3218) (21.8016, -47.3407) (21.8232, -47.3592) (21.845, -47.3775) (21.867, -47.3957) (21.8891, -47.4138) (21.9113, -47.4317) (21.9338, -47.4494) (21.9566, -47.4668) (21.9797, -47.4839) (22.003, -47.5008) (22.0265, -47.5175) (22.0503, -47.534) (22.0741, -47.5503) (22.0982, -47.5665) (22.1224, -47.5825) (22.1467, -47.5984) (22.1712, -47.6141) (22.1959, -47.6297) (22.2207, -47.645) (22.2457, -47.6602) (22.2709, -47.6753) (22.2962, -47.6902) (22.3216, -47.7049) (22.3472, -47.7195) (22.3729, -47.7339) (22.3987, -47.7483) (22.4247, -47.7624) (22.4508, -47.7764) (22.477, -47.7903) (22.5033, -47.804) (22.5298, -47.8176) (22.5564, -47.8311) (22.5831, -47.8444) (22.61, -47.8576) (22.6369, -47.8707) (22.664, -47.8836) (22.6912, -47.8964) (22.7185, -47.909) (22.7459, -47.9216) (22.7734, -47.934) (22.801, -47.9462) (22.8287, -47.9584) (22.8565, -47.9704) (22.8845, -47.9823) (22.9125, -47.994) (22.9406, -48.0057) (22.9688, -48.0172) (22.9972, -48.0286) (23.0256, -48.0398) (23.0541, -48.051) (23.0828, -48.062) (23.1115, -48.0729) (23.1403, -48.0837) (23.1692, -48.0943) (23.1982, -48.1048) (23.2273, -48.1152) (23.2564, -48.1255) (23.2857, -48.1357) (23.315, -48.1457) (23.3445, -48.1557) (23.374, -48.1655) (23.4036, -48.1752) (23.4333, -48.1847) (23.4631, -48.1942) (23.493, -48.2035) (23.5169, -48.2109) (23.5349, -48.2164) (23.5469, -48.22) (23.5529, -48.2218) knots 0 0 0 0 0 0 0.01428571 0.02857143 0.04285714 0.05714286 0.07142857 0.08571429 0.1 0.11428571 0.12857143 0.14285714 0.15714286 0.17142857 0.18571429 0.2 0.21428571 0.22857143 0.24285714 0.25714286 0.27142857 0.28571429 0.3 0.31428571 0.32857143 0.34285714 0.35714286 0.37142857 0.38571429 0.4 0.41428571 0.42857143 0.44285714 0.45714286 0.47142857 0.48571429 0.5 0.51428571 0.52857143 0.54285714 0.55714286 0.57142857 0.58571429 0.6 0.61428571 0.62857143 0.64285714 0.65714286 0.67142857 0.68571429 0.7 0.71428571 0.72857143 0.74285714 0.75714286 0.77142857 0.78571429 0.8 0.81428571 0.82857143 0.84285714 0.85714286 0.87142857 0.88571429 0.9 0.91428571 0.92857143 0.94285714 0.95714286 0.97142857 0.98571429 1 1 1 1 1 1
  arc A14 (23.5529, -48.2218) -> (24.1221, -47.6527) centre (13.5, -37.5997) ccw
  spline S7 degree 5 poles (24.1221, -47.6527) (24.1203, -47.6467) (24.1167, -47.6346) (24.1112, -47.6166) (24.1038, -47.5927) (24.0945, -47.5628) (24.085, -47.533) (24.0754, -47.5033) (24.0658, -47.4737) (24.056, -47.4442) (24.046, -47.4148) (24.036, -47.3854) (24.0258, -47.3561) (24.0155, -47.327) (24.0051, -47.2979) (23.9946, -47.2689) (23.9839, -47.24) (23.9732, -47.2112) (23.9623, -47.1825) (23.9513, -47.1538) (23.9401, -47.1253) (23.9289, -47.0969) (23.9175, -47.0686) (23.906, -47.0403) (23.8943, -47.0122) (23.8826, -46.9842) (23.8707, -46.9562) (23.8587, -46.9284) (23.8465, -46.9007) (23.8343, -46.8731) (23.8219, -46.8456) (23.8093, -46.8182) (23.7967, -46.7909) (23.7839, -46.7637) (23.771, -46.7366) (23.7579, -46.7097) (23.7447, -46.6829) (23.7314, -46.6561) (23.7179, -46.6295) (23.7043, -46.6031) (23.6906, -46.5767) (23.6767, -46.5505) (23.6627, -46.5244) (23.6485, -46.4984) (23.6342, -46.4726) (23.6198, -46.4469) (23.6052, -46.4213) (23.5904, -46.3959) (23.5756, -46.3706) (23.5605, -46.3454) (23.5453, -46.3204) (23.53, -46.2956) (23.5144, -46.2709) (23.4987, -46.2464) (23.4828, -46.2221) (23.4668, -46.1979) (23.4506, -46.1739) (23.4343, -46.15) (23.4178, -46.1262) (23.4011, -46.1027) (23.3842, -46.0794) (23.3671, -46.0563) (23.3496, -46.0335) (23.332, -46.011) (23.314, -45.9888) (23.296, -45.9667) (23.2778, -45.9447) (23.2595, -45.9229) (23.241, -45.9013) (23.2221, -45.8801) (23.2028, -45.8594) (23.1867, -45.8436) (23.1742, -45.8321) (23.1656, -45.8247) (23.1613, -45.821) knots -1 -1 -1 -1 -1 -1 -0.98571429 -0.97142857 -0.95714286 -0.94285714 -0.92857143 -0.91428571 -0.9 -0.88571429 -0.87142857 -0.85714286 -0.84285714 -0.82857143 -0.81428571 -0.8 -0.78571429 -0.77142857 -0.75714286 -0.74285714 -0.72857143 -0.71428571 -0.7 -0.68571429 -0.67142857 -0.65714286 -0.64285714 -0.62857143 -0.61428571 -0.6 -0.58571429 -0.57142857 -0.55714286 -0.54285714 -0.52857143 -0.51428571 -0.5 -0.48571429 -0.47142857 -0.45714286 -0.44285714 -0.42857143 -0.41428571 -0.4 -0.38571429 -0.37142857 -0.35714286 -0.34285714 -0.32857143 -0.31428571 -0.3 -0.28571429 -0.27142857 -0.25714286 -0.24285714 -0.22857143 -0.21428571 -0.2 -0.18571429 -0.17142857 -0.15714286 -0.14285714 -0.12857143 -0.11428571 -0.1 -0.08571429 -0.07142857 -0.05714286 -0.04285714 -0.02857143 -0.01428571 0 0 0 0 0 0
  line L7 (23.1613, -45.821) -> (22.8659, -45.5696)
  arc A15 (22.854, -45.4293) -> (22.8659, -45.5696) centre (22.9307, -45.4935) ccw
  arc A16 (22.854, -45.4293) -> (23.4838, -44.6086) centre (13.5, -37.5997) ccw
  arc A17 (23.6224, -44.5837) -> (23.4838, -44.6086) centre (23.5656, -44.666) ccw
  line L8 (23.6224, -44.5837) -> (23.9417, -44.804)
  spline S8 degree 5 poles (23.9417, -44.804) (23.9463, -44.8072) (23.9557, -44.8135) (23.97, -44.8226) (23.9895, -44.8341) (24.0145, -44.8475) (24.0399, -44.8601) (24.0655, -44.8724) (24.0913, -44.8845) (24.1173, -44.8964) (24.1433, -44.9081) (24.1694, -44.9196) (24.1957, -44.9309) (24.2222, -44.9418) (24.249, -44.9524) (24.2758, -44.9627) (24.3029, -44.9727) (24.3301, -44.9825) (24.3574, -44.9921) (24.3848, -45.0015) (24.4123, -45.0108) (24.4399, -45.0198) (24.4677, -45.0286) (24.4955, -45.0373) (24.5235, -45.0457) (24.5516, -45.0539) (24.5798, -45.0619) (24.608, -45.0697) (24.6364, -45.0774) (24.6649, -45.0849) (24.6935, -45.0922) (24.7221, -45.0993) (24.7509, -45.1063) (24.7797, -45.113) (24.8086, -45.1197) (24.8376, -45.1261) (24.8667, -45.1324) (24.8959, -45.1385) (24.9252, -45.1445) (24.9545, -45.1503) (24.9839, -45.1559) (25.0134, -45.1614) (25.043, -45.1667) (25.0726, -45.1719) (25.1023, -45.1769) (25.1321, -45.1817) (25.1619, -45.1864) (25.1918, -45.191) (25.2218, -45.1954) (25.2519, -45.1996) (25.282, -45.2037) (25.3122, -45.2077) (25.3424, -45.2115) (25.3728, -45.2152) (25.4031, -45.2187) (25.4336, -45.2221) (25.4641, -45.2253) (25.4946, -45.2284) (25.5252, -45.2313) (25.5559, -45.2341) (25.5866, -45.2368) (25.6174, -45.2393) (25.6483, -45.2417) (25.6792, -45.244) (25.7101, -45.2461) (25.7411, -45.248) (25.7722, -45.2499) (25.8033, -45.2516) (25.8344, -45.2531) (25.8657, -45.2546) (25.8969, -45.2558) (25.922, -45.2568) (25.9408, -45.2574) (25.9533, -45.2578) (25.9596, -45.258) knots 0 0 0 0 0 0 0.01428571 0.02857143 0.04285714 0.05714286 0.07142857 0.08571429 0.1 0.11428571 0.12857143 0.14285714 0.15714286 0.17142857 0.18571429 0.2 0.21428571 0.22857143 0.24285714 0.25714286 0.27142857 0.28571429 0.3 0.31428571 0.32857143 0.34285714 0.35714286 0.37142857 0.38571429 0.4 0.41428571 0.42857143 0.44285714 0.45714286 0.47142857 0.48571429 0.5 0.51428571 0.52857143 0.54285714 0.55714286 0.57142857 0.58571429 0.6 0.61428571 0.62857143 0.64285714 0.65714286 0.67142857 0.68571429 0.7 0.71428571 0.72857143 0.74285714 0.75714286 0.77142857 0.78571429 0.8 0.81428571 0.82857143 0.84285714 0.85714286 0.87142857 0.88571429 0.9 0.91428571 0.92857143 0.94285714 0.95714286 0.97142857 0.98571429 1 1 1 1 1 1
  arc A18 (25.9596, -45.258) -> (26.362, -44.5609) centre (13.5, -37.5997) ccw
  spline S9 degree 5 poles (26.362, -44.5609) (26.3587, -44.5556) (26.3521, -44.5449) (26.3422, -44.5289) (26.3289, -44.5077) (26.3121, -44.4813) (26.2953, -44.455) (26.2783, -44.4288) (26.2613, -44.4027) (26.2442, -44.3767) (26.227, -44.3508) (26.2097, -44.3251) (26.1923, -44.2994) (26.1748, -44.2739) (26.1572, -44.2485) (26.1396, -44.2232) (26.1218, -44.1981) (26.1039, -44.173) (26.086, -44.1481) (26.0679, -44.1233) (26.0498, -44.0986) (26.0316, -44.0741) (26.0132, -44.0497) (25.9948, -44.0254) (25.9763, -44.0012) (25.9577, -43.9772) (25.939, -43.9533) (25.9202, -43.9295) (25.9012, -43.9059) (25.8822, -43.8824) (25.8632, -43.859) (25.844, -43.8358) (25.8247, -43.8127) (25.8053, -43.7898) (25.7858, -43.767) (25.7662, -43.7443) (25.7465, -43.7218) (25.7267, -43.6995) (25.7069, -43.6773) (25.6869, -43.6552) (25.6668, -43.6333) (25.6466, -43.6116) (25.6263, -43.59) (25.6059, -43.5686) (25.5854, -43.5473) (25.5648, -43.5262) (25.5441, -43.5053) (25.5232, -43.4846) (25.5023, -43.464) (25.4813, -43.4436) (25.4601, -43.4234) (25.4389, -43.4033) (25.4175, -43.3835) (25.3959, -43.3639) (25.3743, -43.3445) (25.3526, -43.3253) (25.3307, -43.3063) (25.3087, -43.2874) (25.2867, -43.2688) (25.2645, -43.2504) (25.2421, -43.2322) (25.2196, -43.2144) (25.1969, -43.1969) (25.174, -43.1797) (25.1509, -43.1629) (25.1277, -43.1462) (25.1045, -43.1297) (25.0811, -43.1134) (25.0577, -43.0973) (25.034, -43.0817) (25.0099, -43.0667) (24.9903, -43.0556) (24.9752, -43.0477) (24.9651, -43.0428) (24.96, -43.0403) knots -1 -1 -1 -1 -1 -1 -0.98571429 -0.97142857 -0.95714286 -0.94285714 -0.92857143 -0.91428571 -0.9 -0.88571429 -0.87142857 -0.85714286 -0.84285714 -0.82857143 -0.81428571 -0.8 -0.78571429 -0.77142857 -0.75714286 -0.74285714 -0.72857143 -0.71428571 -0.7 -0.68571429 -0.67142857 -0.65714286 -0.64285714 -0.62857143 -0.61428571 -0.6 -0.58571429 -0.57142857 -0.55714286 -0.54285714 -0.52857143 -0.51428571 -0.5 -0.48571429 -0.47142857 -0.45714286 -0.44285714 -0.42857143 -0.41428571 -0.4 -0.38571429 -0.37142857 -0.35714286 -0.34285714 -0.32857143 -0.31428571 -0.3 -0.28571429 -0.27142857 -0.25714286 -0.24285714 -0.22857143 -0.21428571 -0.2 -0.18571429 -0.17142857 -0.15714286 -0.14285714 -0.12857143 -0.11428571 -0.1 -0.08571429 -0.07142857 -0.05714286 -0.04285714 -0.02857143 -0.01428571 0 0 0 0 0 0
  line L9 (24.96, -43.0403) -> (24.6096, -42.874)
  arc A19 (24.5618, -42.7415) -> (24.6096, -42.874) centre (24.6524, -42.7836) ccw
  arc A20 (24.5618, -42.7415) -> (24.9576, -41.7858) centre (13.5, -37.5997) ccw
  arc A21 (25.0851, -41.7259) -> (24.9576, -41.7858) centre (25.0516, -41.8201) ccw
  line L10 (25.0851, -41.7259) -> (25.4505, -41.856)
  spline S10 degree 5 poles (25.4505, -41.856) (25.4558, -41.8579) (25.4665, -41.8616) (25.4827, -41.8667) (25.5045, -41.8727) (25.5321, -41.8791) (25.5599, -41.8848) (25.5878, -41.89) (25.6159, -41.895) (25.644, -41.8998) (25.6722, -41.9044) (25.7004, -41.9088) (25.7287, -41.9128) (25.7572, -41.9165) (25.7857, -41.9199) (25.8144, -41.9228) (25.8431, -41.9255) (25.8719, -41.9279) (25.9007, -41.9301) (25.9296, -41.9321) (25.9586, -41.9339) (25.9876, -41.9355) (26.0167, -41.9369) (26.0458, -41.938) (26.075, -41.9389) (26.1043, -41.9395) (26.1336, -41.94) (26.1629, -41.9402) (26.1923, -41.9403) (26.2218, -41.9401) (26.2512, -41.9398) (26.2808, -41.9393) (26.3103, -41.9385) (26.34, -41.9376) (26.3696, -41.9365) (26.3993, -41.9353) (26.429, -41.9338) (26.4588, -41.9321) (26.4886, -41.9303) (26.5184, -41.9283) (26.5483, -41.9262) (26.5782, -41.9238) (26.6081, -41.9213) (26.6381, -41.9186) (26.6681, -41.9158) (26.6981, -41.9128) (26.7281, -41.9096) (26.7582, -41.9062) (26.7883, -41.9027) (26.8185, -41.8991) (26.8486, -41.8952) (26.8788, -41.8912) (26.909, -41.8871) (26.9392, -41.8828) (26.9695, -41.8783) (26.9998, -41.8737) (27.03, -41.8689) (27.0604, -41.864) (27.0907, -41.8589) (27.1211, -41.8537) (27.1514, -41.8483) (27.1818, -41.8428) (27.2122, -41.8371) (27.2427, -41.8313) (27.2731, -41.8253) (27.3036, -41.8192) (27.334, -41.8129) (27.3645, -41.8065) (27.395, -41.8) (27.4255, -41.7933) (27.4561, -41.7864) (27.4805, -41.7808) (27.4988, -41.7766) (27.511, -41.7737) (27.5172, -41.7722) knots 0 0 0 0 0 0 0.01428571 0.02857143 0.04285714 0.05714286 0.07142857 0.08571429 0.1 0.11428571 0.12857143 0.14285714 0.15714286 0.17142857 0.18571429 0.2 0.21428571 0.22857143 0.24285714 0.25714286 0.27142857 0.28571429 0.3 0.31428571 0.32857143 0.34285714 0.35714286 0.37142857 0.38571429 0.4 0.41428571 0.42857143 0.44285714 0.45714286 0.47142857 0.48571429 0.5 0.51428571 0.52857143 0.54285714 0.55714286 0.57142857 0.58571429 0.6 0.61428571 0.62857143 0.64285714 0.65714286 0.67142857 0.68571429 0.7 0.71428571 0.72857143 0.74285714 0.75714286 0.77142857 0.78571429 0.8 0.81428571 0.82857143 0.84285714 0.85714286 0.87142857 0.88571429 0.9 0.91428571 0.92857143 0.94285714 0.95714286 0.97142857 0.98571429 1 1 1 1 1 1